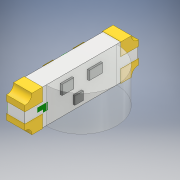
# Autodesk Inventor part: LED 3216 RA
Saved by Autodesk Inventor 2018 (Build 220112000, 112)
## iProperties
Created: 2018-02-20
Part Number: LED 3216 RA
Material: Generic
Document SubType Name: Modeling
Designer: danil
Density: 1 g/cm^3
Appearance: Generic
Author: danil
Autodesk Inventor part; units mm, degrees
ref_plane "YZ Plane" through (0, 0, 0) normal (1, 0, 0) x (0, 1, 0)
ref_plane "XZ Plane" through (0, 0, 0) normal (0, 1, 0) x (-1, 0, 0)
ref_plane "XY Plane" through (0, 0, 0) normal (0, 0, 1) x (1, 0, 0)
sketch "Sketch1" plane through (0, 0, 0) normal (0, 0, 1) x (1, 0, 0)
  arc A0 (0, -1) -> (0, 1) centre (0, 0) ccw
  line L0 (0, 0) -> (0, 1) construction
  line L1 (0, 0) -> (1, 0) construction
  line L2 (0, 0) -> (0, -1) construction
  line L3 (0, 1) -> (0, -1)
  dimension "d0" = 1
  dimension "d1" = 90
  dimension "d2" = 180
  constraints: 8 end point, 2 point on circle, 1 centre point, 1 coincident, 1 horizontal, 1 perpendicular
  measures "d0" radius of A0
  measures "d1" angle of L1 L0
  measures "d2" angle of L2 L0
extrude "Extrusion1" add sketch "Sketch1" along normal blind 1
sketch "Sketch2" plane through (0, -1, 0) normal (-1, 0, 0) x (0, 0, 1)
  line L0 (0, 2.6) -> (1, 2.6)
  line L1 (1, 2.6) -> (1, -0.6)
  line L2 (1, -0.6) -> (0, -0.6)
  line L3 (0, -0.6) -> (0, 2.6)
  line L4 (0, 2) -> (0, 0) projected
  line L5 (1, 2) -> (1, 0) projected
  arc A0 (0, 2.4) -> (0.2, 2.6) centre (0, 2.6) ccw
  arc A1 (0.8, 2.6) -> (1, 2.4) centre (1, 2.6) ccw
  arc A2 (1, -0.4) -> (0.8, -0.6) centre (1, -0.6) ccw
  arc A3 (0.2, -0.6) -> (0, -0.4) centre (0, -0.6) ccw
  point P0 (0, 1)
  point P1 (1, 1)
  point P2 (1, 1)
  dimension "d5" = 3.2
  dimension "d6" = 0.2
  constraints: 8 end point, 8 point on circle, 8 point on line, 5 coincident, 4 centre point, 3 equal radius, 2 collinear, 2 midpoint, 2 parallel, 1 horizontal, 1 perpendicular
  measures "d5" distance of L2.end L0.start
  measures "d6" radius of A0
extrude "Extrusion2" add sketch "Sketch2" along normal blind 0.5 separate body contours L0 A1 L1 A2 L2 A3 L3 A0
sketch "Sketch3" plane through (-0.5, -1, 0) normal (-1, 0, 0) x (0, 0, 1)
  line L0 (0, 2.4) -> (0, -0.4) construction
  arc A0 (0.2, -0.6) -> (0, -0.4) centre (0, -0.6) ccw projected
  line L1 (0.2, -0.6) -> (0.8, -0.6) projected
  arc A1 (1, -0.4) -> (0.8, -0.6) centre (1, -0.6) ccw projected
  line L2 (1, -0.4) -> (1, 2.4) construction
  arc A2 (0.8, 2.6) -> (1, 2.4) centre (1, 2.6) ccw projected
  line L3 (0.8, 2.6) -> (0.2, 2.6) projected
  arc A3 (0, 2.4) -> (0.2, 2.6) centre (0, 2.6) ccw projected
  line L4 (1.01, 2.4103) -> (1.01, -0.4103)
  arc A4 (1.01, -0.4103) -> (0.8103, -0.61) centre (1, -0.6) ccw
  line L5 (0.8103, -0.61) -> (0.1897, -0.61)
  arc A5 (0.1897, -0.61) -> (-0.01, -0.4103) centre (0, -0.6) ccw
  line L6 (-0.01, -0.4103) -> (-0.01, 2.4103)
  arc A6 (-0.01, 2.4103) -> (0.1897, 2.61) centre (0, 2.6) ccw
  line L7 (0.1897, 2.61) -> (0.8103, 2.61)
  arc A7 (0.8103, 2.61) -> (1.01, 2.4103) centre (1, 2.6) ccw
  line L8 (-0.01, 2.11) -> (1.01, 2.11)
  line L9 (-0.01, -0.11) -> (1.01, -0.11)
  line L10 (0.35, -0.61) -> (0.35, -0.11)
  line L11 (0.65, -0.61) -> (0.65, -0.11)
  line L12 (0.35, 2.11) -> (0.35, 2.61)
  line L13 (0.65, 2.11) -> (0.65, 2.61)
  line L14 (-0.01, 0.39) -> (1.01, 0.39)
  line L15 (1.01, 0.39) -> (1.01, 0.79)
  line L16 (1.01, 0.79) -> (-0.01, 0.79)
  line L17 (-0.01, 0.79) -> (-0.01, 0.39)
  line L18 (-0.01, 1.21) -> (1.01, 1.21)
  line L19 (1.01, 1.21) -> (1.01, 1.61)
  line L20 (1.01, 1.61) -> (-0.01, 1.61)
  line L21 (-0.01, 1.61) -> (-0.01, 1.21)
  line L22 (0.3264, 0.39) -> (0.3264, 0.6716)
  line L23 (0.3264, 0.6716) -> (1, 0.6716)
  line L24 (1, 0) -> (1, 2) projected
  line L25 (0.7999, 0.39) -> (0.7999, -0.11)
  line L26 (0.8988, -0.11) -> (0.8988, 0.39)
  line L27 (0.8988, 0.6716) -> (0.8988, 0.6093)
  line L28 (0.8988, 0.6093) -> (1.01, 0.6093)
  line L29 (0.8988, 1.21) -> (0.8988, 1.2723)
  line L30 (0.8988, 1.2723) -> (1.01, 1.2723)
  line L31 (0.8988, 0.39) -> (0.8988, 0.4202)
  line L32 (0.8988, 0.4202) -> (1.01, 0.4202)
  line L33 (0.8988, 1.61) -> (0.8988, 1.5798)
  line L34 (0.8988, 1.5798) -> (1.01, 1.5798)
  line L35 (0.8988, 1.61) -> (0.8988, 1.6766)
  line L36 (0.8988, 1.6766) -> (0.8988, 2.11)
  line L37 (0.7999, 2.11) -> (0.7999, 1.61)
  line L38 (0.3264, 1.21) -> (0.3264, 1.4376)
  line L39 (0.3264, 1.4376) -> (0.7999, 1.4376)
  line L40 (0.7999, 1.4376) -> (0.7999, 1.21)
  line L41 (0.7999, 1.2723) -> (0.8988, 1.2723)
  line L42 (0.7999, 0.39) -> (0.7999, 0.6716)
  line L43 (0.8988, 0.79) -> (0.8988, 0.7073)
  line L44 (0.8988, 0.7073) -> (1.01, 0.7073)
  dimension "d9" = 0.01
  dimension "d10" = 0.5
  dimension "d11" = 0.5
  dimension "d23" = 0.35
  dimension "d24" = 0.35
  dimension "d25" = 0.4
  dimension "d26" = 0.4
  dimension "d27" = 0.5
  dimension "d28" = 0.5
  constraints: 80 end point, 41 point on line, 21 perpendicular, 8 collinear, 8 point on circle, 5 vertical, 4 centre point, 4 parallel, 2 horizontal, 7 other
  measures "d9" radial gap between concentric circles of A2 A7
  measures "d10" distance between parallel lines of L5 L9
  measures "d11" distance between parallel lines of L8 L7
  measures "d23" distance between parallel lines of L0 L10
  measures "d24" distance between parallel lines of L2 L11
  measures "d25" distance between parallel lines of L16 L14
  measures "d26" distance between parallel lines of L20 L18
  measures "d27" distance between parallel lines of L14 L9
  measures "d28" distance between parallel lines of L20 L8
extrude "Extrusion4" add sketch "Sketch3" along normal blind 0.01 separate body contours L10 L5 A5 L6 L9 | L11 L9 L4 A4 L5 | L25 L14 L26 L9 | L6 L16 L43 L44 L24 L23 L22 L14 | L42 L23 L27 L28 L24 L32 L31 L14 | L6 L20 L33 L34 L24 L30 L41 L40 L39 L38 L18 | L23 L24 L28 L27 | L32 L24 L28 L4 | L24 L44 L4 L28 | L6 A6 L7 L12 L8 | L37 L8 L36 L35 L20 | L8 L13 L7 A7 L4 | L24 L34 L4 L30
extrude "Extrusion8" add sketch "Sketch3" against normal blind 0.51 contours L10 L5 A5 L6 L9 | L11 L9 L4 A4 L5 | L6 A6 L7 L12 L8 | L8 L13 L7 A7 L4 bodies 3
sketch "Sketch4" plane through (-0.5, -1, 0) normal (-1, 0, 0) x (0, 0, 1)
  line L0 (1, -0.4) -> (1, 2.4) projected
  line L1 (1, 0) -> (1, 2) projected
  line L2 (1, 0.9206) -> (0, 0.9206)
  line L3 (0, 0.9206) -> (0, 1.0913)
  line L4 (0, 1.0913) -> (1, 1.0913)
  line L5 (1, 1.0913) -> (1, 0.9206)
  line L6 (0, 2.4) -> (0, -0.4) projected
  line L7 (0, 0) -> (0, 2) projected
  line L8 (0, 2) -> (1, 2) projected
  line L9 (0, 1.7644) -> (0.3326, 1.7644)
  line L10 (0.3326, 1.7644) -> (0.3326, 2)
  line L11 (0.3326, 2) -> (0, 2)
  line L12 (0, 2) -> (0, 1.7644)
  line L13 (0, 2.4) -> (0, -0.4) projected
  line L14 (0, 0.0646) -> (0.5437, 0.0646)
  line L15 (0.5437, 0.0646) -> (0.5437, 0.2502)
  line L16 (0.5437, 0.2502) -> (0, 0.2502)
  line L17 (0, 0.2502) -> (0, 0.0646)
  line L18 (0.426, -0.6) -> (0.5728, -0.6)
  line L19 (0.5728, -0.6) -> (0.5728, 0.5851)
  line L20 (0.5728, 0.5851) -> (0.426, 0.5851)
  line L21 (0.426, 0.5851) -> (0.426, -0.6)
  line L22 (0.2, -0.6) -> (0.8, -0.6) projected
  point P0 (0, 1)
  point P1 (1, 1.9835)
  constraints: 32 end point, 8 parallel, 4 horizontal, 4 perpendicular, 4 point on line, 2 collinear, 2 other
extrude "Extrusion5" add sketch "Sketch4" along normal blind 0.001 separate body contours L2 L3 L4 L0 | L16 L21 L14 L6 | L10 L9 L6 L8 | L21 L20 L19 L18 L14 L15 L16 | L16 L15 L14 L21
sketch "Sketch5" plane through (0, -1, 0) normal (1, 0, 0) x (0, 0, -1)
  line L0 (-0.447, -0.2461) -> (-0.5616, -0.2461)
  line L1 (-0.5616, -0.2461) -> (-0.5616, 0.0527)
  line L2 (-0.5616, 0.0527) -> (-0.3686, 0.0527)
  line L3 (-0.3686, 0.0527) -> (-0.3686, -0.0817)
  line L4 (-0.3686, -0.0817) -> (-0.447, -0.0817)
  line L5 (-0.447, -0.0817) -> (-0.447, -0.2461)
  constraints: 12 end point, 5 perpendicular, 1 horizontal
extrude "Extrusion6" add sketch "Sketch5" along normal blind 0.001 bodies 4
sketch "Sketch6" plane through (0, -1, 0) normal (1, 0, 0) x (0, 0, -1)
  line L0 (-0.8383, 0.4024) -> (-0.5632, 0.4024)
  line L1 (-0.5632, 0.4024) -> (-0.5632, 0.7349)
  line L2 (-0.5632, 0.7349) -> (-0.8383, 0.7349)
  line L3 (-0.8383, 0.7349) -> (-0.8383, 0.4024)
  line L4 (-0.7989, 1.1723) -> (-0.5452, 1.1723)
  line L5 (-0.5452, 1.1723) -> (-0.5452, 1.5529)
  line L6 (-0.5452, 1.5529) -> (-0.7989, 1.5529)
  line L7 (-0.7989, 1.5529) -> (-0.7989, 1.1723)
  line L8 (-0.3746, 0.7655) -> (-0.1428, 0.7655)
  line L9 (-0.1428, 0.7655) -> (-0.1428, 1.0105)
  line L10 (-0.1428, 1.0105) -> (-0.3746, 1.0105)
  line L11 (-0.3746, 1.0105) -> (-0.3746, 0.7655)
  point P0 (0, 1)
  constraints: 24 end point, 6 parallel, 3 horizontal, 3 perpendicular
extrude "Extrusion7" add sketch "Sketch6" along normal blind 0.05 separate body
equation "\"d11\" = d10"
equation "\"d24\" = d23"
equation "\"d26\" = d25"
body "Solid1"
body "Solid2"
body "Solid4"
body "Solid5"
body "Solid6"
